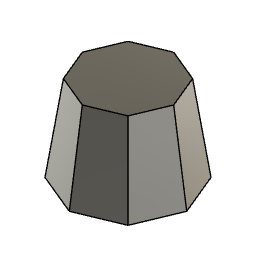
blender-01 v6 (Autodesk Fusion 360 design; units mm, degrees)
Autodesk Fusion 360 part; units mm, degrees
sketch "Sketch1" plane through (0, 0, 0) normal (0, 0, 1) x (1, 0, 0) in component "boiler"
  line L0 (38.8029, -38.8029) -> (54.8756, 0)
  line L1 (54.8756, 0) -> (38.8029, 38.8029)
  line L2 (38.8029, 38.8029) -> (0, 54.8756)
  line L3 (0, 54.8756) -> (-38.8029, 38.8029)
  line L4 (-38.8029, 38.8029) -> (-54.8756, 0)
  line L5 (-54.8756, 0) -> (-38.8029, -38.8029)
  line L6 (-38.8029, -38.8029) -> (0, -54.8756)
  line L7 (0, -54.8756) -> (38.8029, -38.8029)
  line L8 (0, 0) -> (0, -54.8756) construction
  dimension "d1" = 42
  constraint coincident L8.start origin
  constraint vertical L8
  constraint coincident L6.end L7.start
  measures "d1" distance of L0.start L6.end
extrude "Extrude1" add sketch "Sketch1" along normal blind 80 draft -8 in component "boiler"
component "boiler" placed x (1, 0, 0) y (0, 1, 0) z (0, 0, 1) at (0, 0, 0)
